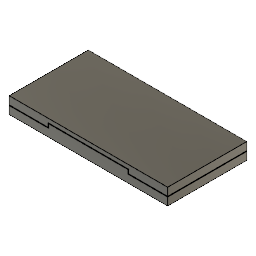
4.7 parameters (Autodesk Fusion 360 design; units mm, degrees)
Autodesk Fusion 360 part; units mm, degrees
sketch "Sketch2" plane through (0, 0, 0) normal (0, 0, 1) x (1, 0, 0)
  line L0 (0, 0) -> (60, 0)
  line L1 (60, 0) -> (60, 30)
  line L2 (60, 30) -> (0, 30)
  line L3 (0, 30) -> (0, 0)
  dimension "d8" = 60
  dimension "d9" = 30
  constraint horizontal L0
  constraint vertical L1
  constraint horizontal L2
  constraint vertical L3
  constraint coincident L0.start L3.end
  measures "d8" distance of L1.end L2.end
  measures "d9" distance of L0.end L1.end
extrude "Extrude5" add sketch "Sketch2" along normal blind 3 makes body 1
sketch "Sketch6" plane through (0, 0, 0) normal (0, 1, 0) x (1, 0, 0)
  line L0 (45, -4.5) -> (15, -4.5)
  line L1 (15, -4.5) -> (15, -1.5)
  line L2 (15, -1.5) -> (45, -1.5)
  line L3 (45, -1.5) -> (45, -4.5)
  line L4 (45, -4.5) -> (15, -1.5) construction
  line L5 (15, -4.5) -> (45, -1.5) construction
  line L6 (0, -3) -> (60, -3)
  point P0 (30, -3)
  dimension "d36" = 30
  dimension "d37" = 3
  constraint perpendicular L0 L1
  constraint parallel L0 L2
  constraint parallel L1 L3
  constraint horizontal L0
  constraint coincident L4 P0
  constraint coincident L5 P0
  constraint midpoint P0 L6
  measures "d36" distance of L0.start L0.end
  measures "d37" distance of L0.start L2.end
extrude "Extrude6" add sketch "Sketch6" along normal blind 30 contours L0 L1 L3 L6 bodies 1
ref_plane "WorkPlane2" through (0, 0, 3.2) normal (0, 0, 1) x (1, 0, 0)
sketch "Sketch7" plane through (0, 0, 3.2) normal (0, 0, 1) x (1, 0, 0)
  line L0 (0, 0) -> (60, 0)
  line L1 (60, 0) -> (60, 30)
  line L2 (60, 30) -> (0, 30)
  line L3 (0, 30) -> (0, 0)
  dimension "d41" = 60
  dimension "d42" = 30
  constraint horizontal L0
  constraint vertical L1
  constraint horizontal L2
  constraint vertical L3
  constraint coincident L0.start L3.end
  measures "d41" distance of L1.end L2.end
  measures "d42" distance of L0.end L1.end
extrude "Extrude7" add sketch "Sketch7" along normal blind 3 separate body makes body 2
sketch "Sketch8" plane through (0, 0, 0) normal (0, 1, 0) x (1, 0, 0)
  line L0 (45.2, -1.7) -> (14.8, -1.7)
  line L1 (14.8, -1.7) -> (14.8, -4.7)
  line L2 (14.8, -4.7) -> (45.2, -4.7)
  line L3 (45.2, -4.7) -> (45.2, -1.7)
  line L4 (45.2, -1.7) -> (14.8, -4.7) construction
  line L5 (14.8, -1.7) -> (45.2, -4.7) construction
  line L6 (0, -3.2) -> (60, -3.2)
  point P0 (30, -3.2)
  dimension "d45" = 30.4
  dimension "d46" = 3
  constraint perpendicular L0 L1
  constraint parallel L0 L2
  constraint parallel L1 L3
  constraint horizontal L0
  constraint coincident L4 P0
  constraint coincident L5 P0
  constraint midpoint P0 L6
  measures "d45" distance of L1.end L2.end
  measures "d46" distance of L0.start L2.end
extrude "Extrude8" cut sketch "Sketch8" along normal blind 30 contours L1 L2 L3 L6 bodies 2
equation "platelength = 60 mm"
equation "platewidth = 30 mm"
equation "plateheight = 3 mm"
equation "clearence = 0.2 mm"
equation "d8 = platelength"
equation "d9 = platewidth"
equation "d34 = plateheight"
equation "d37 = plateheight"
equation "d38 = platewidth"
equation "d40 = plateheight + clearence"
equation "d41 = platelength"
equation "d42 = platewidth"
equation "d43 = plateheight"
equation "d45 = 30 mm + ( 2 * clearence )"
equation "d46 = plateheight"
equation "d47 = platewidth"
